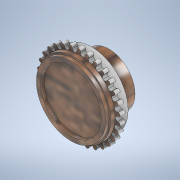
# Autodesk Inventor part: velke_koleso
Saved by Autodesk Inventor 2022 (Build 260153000, 153)
## iProperties
Created: 2021-12-16
Part Number: velke_koleso
Material: Generic
Document SubType Name: Modeling
Designer: MatusBarany
Density: 1 g/cm^3
Appearance: Default
Author: MatusBarany
Autodesk Inventor part; units mm, degrees
ref_plane "YZ Plane" through (0, 0, 0) normal (1, 0, 0) x (0, 1, 0)
ref_plane "XZ Plane" through (0, 0, 0) normal (0, 1, 0) x (-1, 0, 0)
ref_plane "XY Plane" through (0, 0, 0) normal (0, 0, 1) x (1, 0, 0)
sketch "Sketch1" plane through (0, 0, 0) normal (0, 0, 1) x (1, 0, 0)
  circle A0 centre (0, 0) radius 21
  dimension "d0" = 42
  constraints: 1 centre point, 1 coincident
  measures "d0" diameter of A0
extrude "Extrusion1" add sketch "Sketch1" along normal blind 10
sketch "Sketch2" plane through (0, 0, 10) normal (0, 0, 1) x (1, 0, 0)
  circle A0 centre (0, 0) radius 20
  circle A1 centre (0, 0) radius 21 projected
  circle A2 centre (0, 0) radius 17.5
  dimension "d3" = 40
  dimension "d4" = 42
  dimension "d5" = 35
  constraints: 2 centre point, 2 coincident
  measures "d3" diameter of A0
  measures "d4" diameter of A1
  measures "d5" diameter of A2
extrude "Extrusion2" add sketch "Sketch2" along normal blind 2 contours A0
ref_plane "Work Plane1" through (0, 0, 6) normal (0, 0, 1) x (1, 0, 0)
sketch "Sketch3" plane through (0, 0, 6) normal (0, 0, 1) x (1, 0, 0)
  circle A0 centre (0, 0) radius 21 projected
  line L0 (0, 24) -> (0, 21)
  line L1 (0, -30.2358) -> (0, 34.4151) projected
  arc A1 (1, 23) -> (0, 24) centre (0, 23) ccw
  circle A2 centre (0, 0) radius 21 projected
  line L2 (1, 23) -> (1, 22.3607)
  arc A3 (1, 22.3607) -> (2.3333, 20.87) centre (2.5, 22.3607) ccw
  arc A4 (0, 24) -> (-1, 23) centre (0, 23) ccw
  line L3 (-1, 23) -> (-1, 22.3607)
  arc A5 (-2.3333, 20.87) -> (-1, 22.3607) centre (-2.5, 22.3607) ccw
  point P0 (-1.5546, 20.9424)
  dimension "d15" = 3
  dimension "d26" = 1
  dimension "d27" = 90
  dimension "d30" = 0
  dimension "d32" = 1.5
  constraints: 10 point on circle, 6 end point, 4 centre point, 4 symmetric about line, 2 point on line, 2 tangent, 1 vertical, 3 other
  measures "d15" distance of L0.start L0.end
  measures "d26" radius of A1
  measures "d30" distance from line of A0.centre L0
  measures "d32" radius of A3
extrude "Extrusion3" add sketch "Sketch3" along normal mid plane 3
pattern_circular "Circular Pattern1" count 30 over 360 about axis through (0, 0, -10) along (0, 0, 1) of "Extrusion3"
sketch "Sketch4" plane through (0, 0, 0) normal (0, 0, -1) x (-1, 0, 0)
  circle A0 centre (0, 0) radius 17.5 projected
  circle A1 centre (0, 0) radius 15
  arc A2 (-7.5, 8.0467) -> (7.5, 8.0467) centre (0, 0) ccw
  line L0 (7.5, 8.0467) -> (-7.5, 8.0467)
  dimension "d23" = 22
  dimension "d24" = 30
  dimension "d25" = 15
  constraints: 2 centre point, 2 coincident, 2 end point, 2 point on circle, 1 horizontal
  measures "d23" diameter of A2
  measures "d24" diameter of A1
  measures "d25" distance of L0.start L0.end
extrude "Extrusion4" add sketch "Sketch4" along normal blind 10 contours A1
sketch "Sketch6" plane through (-17.2864, 14.2191, 4.5) normal (-0.6691306, -0.7431448, 0) x (0.7431448, -0.6691306, 0)
  point P0 (22.3607, -4.5)
body "Solid1"
